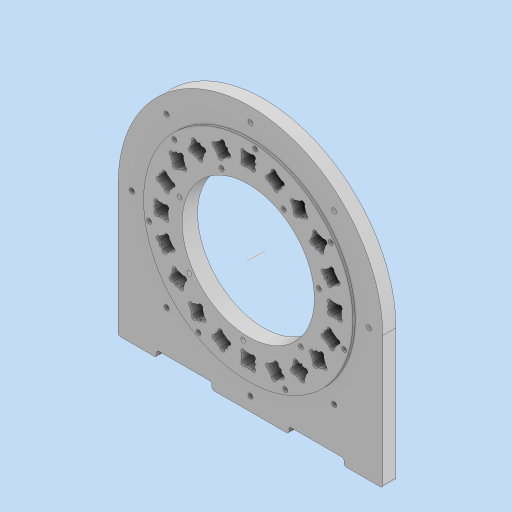
# Autodesk Inventor part: Ring_842
Saved by Autodesk Inventor 2024.2 (Build 282272000, 272)
## iProperties
Created: 2025-04-23
Part Number: Ring_842
Material: Generic
Document SubType Name: Modeling
Designer: 23661194
Density: 1 g/cm^3
Appearance: Default
Author: 23661194
Autodesk Inventor part; units mm, degrees
ref_plane "YZ Plane" through (0, 0, 0) normal (1, 0, 0) x (0, 1, 0)
ref_plane "XZ Plane" through (0, 0, 0) normal (0, 1, 0) x (-1, 0, 0)
ref_plane "XY Plane" through (0, 0, 0) normal (0, 0, 1) x (1, 0, 0)
sketch "Sketch1" plane through (0, 0, 0) normal (0, 0, 1) x (1, 0, 0)
  circle A0 centre (0, 0) radius 60
  circle A1 centre (0, 0) radius 120
  circle A2 centre (0, 0) radius 95
  dimension "d0" = 120
  dimension "d1" = 240
  dimension "d2" = 190
  constraints: 3 centre point, 3 coincident
  measures "d0" diameter of A0
  measures "d1" diameter of A1
  measures "d2" diameter of A2
extrude "Extrusion1" add sketch "Sketch1" along normal blind 12 contours A1 | A2
extrude "Extrusion2" add sketch "Sketch1" along normal blind 14 contours A2
sketch "Sketch3" plane through (0, 0, 14) normal (0, 0, 1) x (1, 0, 0)
  circle A0 centre (0, 0) radius 78.7024
  line L0 (78.7024, 0) -> (0, 0)
  line L1 (74.8504, 24.3204) -> (0, 0)
  line L2 (63.6716, 46.2601) -> (0, 0)
  line L3 (46.2601, 63.6716) -> (0, 0)
  line L4 (24.3204, 74.8504) -> (0, 0)
  line L5 (0, 78.7024) -> (0, 0)
  line L6 (-24.3204, 74.8504) -> (0, 0)
  line L7 (-46.2601, 63.6716) -> (0, 0)
  line L8 (-63.6716, 46.2601) -> (0, 0)
  line L9 (-74.8504, 24.3204) -> (0, 0)
  line L10 (-78.7024, 0) -> (0, 0)
  line L11 (-74.8504, -24.3204) -> (0, 0)
  line L12 (-63.6716, -46.2601) -> (0, 0)
  line L13 (-46.2601, -63.6716) -> (0, 0)
  line L14 (-24.3204, -74.8504) -> (0, 0)
  line L15 (0, -78.7024) -> (0, 0)
  line L16 (24.3204, -74.8504) -> (0, 0)
  line L17 (46.2601, -63.6716) -> (0, 0)
  line L18 (63.6716, -46.2601) -> (0, 0)
  line L19 (74.8504, -24.3204) -> (0, 0)
  line L20 (-168, 0) -> (168, 0) projected
  line L21 (84.6424, 5.94) -> (72.7624, 5.94)
  line L22 (72.7624, 5.94) -> (72.7624, -5.94)
  line L23 (72.7624, -5.94) -> (84.6424, -5.94)
  line L24 (84.6424, -5.94) -> (84.6424, 5.94)
  line L25 (84.6424, 5.94) -> (72.7624, -5.94) construction
  line L26 (72.7624, 5.94) -> (84.6424, -5.94) construction
  circle A1 centre (78.7024, 0) radius 2
  circle A2 centre (74.1754, -4.527) radius 2.1
  circle A3 centre (83.2294, -4.527) radius 2.1
  circle A4 centre (83.2294, 4.527) radius 2.1
  circle A5 centre (74.1754, 4.527) radius 2.1
  circle A6 centre (72.4024, 0) radius 0.75
  line L27 (72.4024, 0) -> (78.7024, 0)
  line L28 (76.1645, 32.6174) -> (66.5534, 25.6345)
  line L29 (66.5534, 25.6345) -> (73.5363, 16.0234)
  line L30 (73.5363, 16.0234) -> (83.1474, 23.0063)
  line L31 (83.1474, 23.0063) -> (76.1645, 32.6174)
  line L32 (76.1645, 32.6174) -> (73.5363, 16.0234) construction
  line L33 (66.5534, 25.6345) -> (83.1474, 23.0063) construction
  circle A7 centre (74.8504, 24.3204) radius 2
  circle A8 centre (73.8489, 17.9971) radius 2.1
  circle A9 centre (81.1737, 23.3189) radius 2.1
  circle A10 centre (75.8519, 30.6437) radius 2.1
  circle A11 centre (68.5271, 25.3219) radius 2.1
  circle A12 centre (69.7536, 20.6173) radius 0.75
  line L34 (69.7536, 20.6173) -> (74.8504, 24.3204)
  line L35 (59.8579, 53.7449) -> (56.1867, 42.4464)
  line L36 (56.1867, 42.4464) -> (67.4853, 38.7753)
  line L37 (67.4853, 38.7753) -> (71.1564, 50.0738)
  line L38 (71.1564, 50.0738) -> (59.8579, 53.7449)
  line L39 (59.8579, 53.7449) -> (67.4853, 38.7753) construction
  line L40 (56.1867, 42.4464) -> (71.1564, 50.0738) construction
  circle A13 centre (63.6716, 46.2601) radius 2
  circle A14 centre (66.5781, 40.5558) radius 2.1
  circle A15 centre (69.3759, 49.1666) radius 2.1
  circle A16 centre (60.7651, 51.9645) radius 2.1
  circle A17 centre (57.9672, 43.3536) radius 2.1
  circle A18 centre (61.7248, 40.2684) radius 0.75
  line L41 (61.7248, 40.2684) -> (63.6716, 46.2601)
  line L42 (38.7753, 67.4853) -> (42.4464, 56.1867)
  line L43 (42.4464, 56.1867) -> (53.7449, 59.8579)
  line L44 (53.7449, 59.8579) -> (50.0738, 71.1564)
  line L45 (50.0738, 71.1564) -> (38.7753, 67.4853)
  line L46 (38.7753, 67.4853) -> (53.7449, 59.8579) construction
  line L47 (42.4464, 56.1867) -> (50.0738, 71.1564) construction
  circle A19 centre (46.2601, 63.6716) radius 2
  circle A20 centre (51.9645, 60.7651) radius 2.1
  circle A21 centre (49.1666, 69.3759) radius 2.1
  circle A22 centre (40.5558, 66.5781) radius 2.1
  circle A23 centre (43.3536, 57.9672) radius 2.1
  circle A24 centre (48.2069, 57.6799) radius 0.75
  line L48 (48.2069, 57.6799) -> (46.2601, 63.6716)
  line L49 (16.0234, 73.5363) -> (25.6345, 66.5534)
  line L50 (25.6345, 66.5534) -> (32.6174, 76.1645)
  line L51 (32.6174, 76.1645) -> (23.0063, 83.1474)
  line L52 (23.0063, 83.1474) -> (16.0234, 73.5363)
  line L53 (16.0234, 73.5363) -> (32.6174, 76.1645) construction
  line L54 (25.6345, 66.5534) -> (23.0063, 83.1474) construction
  circle A25 centre (24.3204, 74.8504) radius 2
  circle A26 centre (30.6437, 75.8519) radius 2.1
  circle A27 centre (23.3189, 81.1737) radius 2.1
  circle A28 centre (17.9971, 73.8489) radius 2.1
  circle A29 centre (25.3219, 68.5271) radius 2.1
  circle A30 centre (29.4172, 71.1474) radius 0.75
  line L55 (29.4172, 71.1474) -> (24.3204, 74.8504)
  line L56 (-5.94, 72.7624) -> (5.94, 72.7624)
  line L57 (5.94, 72.7624) -> (5.94, 84.6424)
  line L58 (5.94, 84.6424) -> (-5.94, 84.6424)
  line L59 (-5.94, 84.6424) -> (-5.94, 72.7624)
  line L60 (-5.94, 72.7624) -> (5.94, 84.6424) construction
  line L61 (5.94, 72.7624) -> (-5.94, 84.6424) construction
  circle A31 centre (0, 78.7024) radius 2
  circle A32 centre (4.527, 83.2294) radius 2.1
  circle A33 centre (-4.527, 83.2294) radius 2.1
  circle A34 centre (-4.527, 74.1754) radius 2.1
  circle A35 centre (4.527, 74.1754) radius 2.1
  circle A36 centre (6.3, 78.7024) radius 0.75
  line L62 (6.3, 78.7024) -> (0, 78.7024)
  line L63 (-25.6345, 66.5534) -> (-16.0234, 73.5363)
  line L64 (-16.0234, 73.5363) -> (-23.0063, 83.1474)
  line L65 (-23.0063, 83.1474) -> (-32.6174, 76.1645)
  line L66 (-32.6174, 76.1645) -> (-25.6345, 66.5534)
  line L67 (-25.6345, 66.5534) -> (-23.0063, 83.1474) construction
  line L68 (-16.0234, 73.5363) -> (-32.6174, 76.1645) construction
  circle A37 centre (-24.3204, 74.8504) radius 2
  circle A38 centre (-23.3189, 81.1737) radius 2.1
  circle A39 centre (-30.6437, 75.8519) radius 2.1
  circle A40 centre (-25.3219, 68.5271) radius 2.1
  circle A41 centre (-17.9971, 73.8489) radius 2.1
  circle A42 centre (-19.2236, 78.5535) radius 0.75
  line L69 (-19.2236, 78.5535) -> (-24.3204, 74.8504)
  line L70 (-42.4464, 56.1867) -> (-38.7753, 67.4853)
  line L71 (-38.7753, 67.4853) -> (-50.0738, 71.1564)
  line L72 (-50.0738, 71.1564) -> (-53.7449, 59.8579)
  line L73 (-53.7449, 59.8579) -> (-42.4464, 56.1867)
  line L74 (-42.4464, 56.1867) -> (-50.0738, 71.1564) construction
  line L75 (-38.7753, 67.4853) -> (-53.7449, 59.8579) construction
  circle A43 centre (-46.2601, 63.6716) radius 2
  circle A44 centre (-49.1666, 69.3759) radius 2.1
  circle A45 centre (-51.9645, 60.7651) radius 2.1
  circle A46 centre (-43.3536, 57.9672) radius 2.1
  circle A47 centre (-40.5558, 66.5781) radius 2.1
  circle A48 centre (-44.3133, 69.6632) radius 0.75
  line L76 (-44.3133, 69.6632) -> (-46.2601, 63.6716)
  line L77 (-56.1867, 42.4464) -> (-59.8579, 53.7449)
  line L78 (-59.8579, 53.7449) -> (-71.1564, 50.0738)
  line L79 (-71.1564, 50.0738) -> (-67.4853, 38.7753)
  line L80 (-67.4853, 38.7753) -> (-56.1867, 42.4464)
  line L81 (-56.1867, 42.4464) -> (-71.1564, 50.0738) construction
  line L82 (-59.8579, 53.7449) -> (-67.4853, 38.7753) construction
  circle A49 centre (-63.6716, 46.2601) radius 2
  circle A50 centre (-69.3759, 49.1666) radius 2.1
  circle A51 centre (-66.5781, 40.5558) radius 2.1
  circle A52 centre (-57.9672, 43.3536) radius 2.1
  circle A53 centre (-60.7651, 51.9645) radius 2.1
  circle A54 centre (-65.6184, 52.2518) radius 0.75
  line L83 (-65.6184, 52.2518) -> (-63.6716, 46.2601)
  line L84 (-66.5534, 25.6345) -> (-76.1645, 32.6174)
  line L85 (-76.1645, 32.6174) -> (-83.1474, 23.0063)
  line L86 (-83.1474, 23.0063) -> (-73.5363, 16.0234)
  line L87 (-73.5363, 16.0234) -> (-66.5534, 25.6345)
  line L88 (-66.5534, 25.6345) -> (-83.1474, 23.0063) construction
  line L89 (-76.1645, 32.6174) -> (-73.5363, 16.0234) construction
  circle A55 centre (-74.8504, 24.3204) radius 2
  circle A56 centre (-81.1737, 23.3189) radius 2.1
  circle A57 centre (-73.8489, 17.9971) radius 2.1
  circle A58 centre (-68.5271, 25.3219) radius 2.1
  circle A59 centre (-75.8519, 30.6437) radius 2.1
  circle A60 centre (-79.9472, 28.0234) radius 0.75
  line L90 (-79.9472, 28.0234) -> (-74.8504, 24.3204)
  line L91 (-72.7624, 5.94) -> (-84.6424, 5.94)
  line L92 (-84.6424, 5.94) -> (-84.6424, -5.94)
  line L93 (-84.6424, -5.94) -> (-72.7624, -5.94)
  line L94 (-72.7624, -5.94) -> (-72.7624, 5.94)
  line L95 (-72.7624, 5.94) -> (-84.6424, -5.94) construction
  line L96 (-84.6424, 5.94) -> (-72.7624, -5.94) construction
  circle A61 centre (-78.7024, 0) radius 2
  circle A62 centre (-83.2294, -4.527) radius 2.1
  circle A63 centre (-74.1754, -4.527) radius 2.1
  circle A64 centre (-74.1754, 4.527) radius 2.1
  circle A65 centre (-83.2294, 4.527) radius 2.1
  circle A66 centre (-85.0024, 0) radius 0.75
  line L97 (-85.0024, 0) -> (-78.7024, 0)
  line L98 (-73.5363, -16.0234) -> (-83.1474, -23.0063)
  line L99 (-83.1474, -23.0063) -> (-76.1645, -32.6174)
  line L100 (-76.1645, -32.6174) -> (-66.5534, -25.6345)
  line L101 (-66.5534, -25.6345) -> (-73.5363, -16.0234)
  line L102 (-73.5363, -16.0234) -> (-76.1645, -32.6174) construction
  line L103 (-83.1474, -23.0063) -> (-66.5534, -25.6345) construction
  circle A67 centre (-74.8504, -24.3204) radius 2
  circle A68 centre (-75.8519, -30.6437) radius 2.1
  circle A69 centre (-68.5271, -25.3219) radius 2.1
  circle A70 centre (-73.8489, -17.9971) radius 2.1
  circle A71 centre (-81.1737, -23.3189) radius 2.1
  circle A72 centre (-79.9472, -28.0234) radius 0.75
  line L104 (-79.9472, -28.0234) -> (-74.8504, -24.3204)
  line L105 (-67.4853, -38.7753) -> (-71.1564, -50.0738)
  line L106 (-71.1564, -50.0738) -> (-59.8579, -53.7449)
  line L107 (-59.8579, -53.7449) -> (-56.1867, -42.4464)
  line L108 (-56.1867, -42.4464) -> (-67.4853, -38.7753)
  line L109 (-67.4853, -38.7753) -> (-59.8579, -53.7449) construction
  line L110 (-71.1564, -50.0738) -> (-56.1867, -42.4464) construction
  circle A73 centre (-63.6716, -46.2601) radius 2
  circle A74 centre (-60.7651, -51.9645) radius 2.1
  circle A75 centre (-57.9672, -43.3536) radius 2.1
  circle A76 centre (-66.5781, -40.5558) radius 2.1
  circle A77 centre (-69.3759, -49.1666) radius 2.1
  circle A78 centre (-65.6184, -52.2518) radius 0.75
  line L111 (-65.6184, -52.2518) -> (-63.6716, -46.2601)
  line L112 (-53.7449, -59.8579) -> (-50.0738, -71.1564)
  line L113 (-50.0738, -71.1564) -> (-38.7753, -67.4853)
  line L114 (-38.7753, -67.4853) -> (-42.4464, -56.1867)
  line L115 (-42.4464, -56.1867) -> (-53.7449, -59.8579)
  line L116 (-53.7449, -59.8579) -> (-38.7753, -67.4853) construction
  line L117 (-50.0738, -71.1564) -> (-42.4464, -56.1867) construction
  circle A79 centre (-46.2601, -63.6716) radius 2
  circle A80 centre (-40.5558, -66.5781) radius 2.1
  circle A81 centre (-43.3536, -57.9672) radius 2.1
  circle A82 centre (-51.9645, -60.7651) radius 2.1
  circle A83 centre (-49.1666, -69.3759) radius 2.1
  circle A84 centre (-44.3133, -69.6632) radius 0.75
  line L118 (-44.3133, -69.6632) -> (-46.2601, -63.6716)
  line L119 (-32.6174, -76.1645) -> (-23.0063, -83.1474)
  line L120 (-23.0063, -83.1474) -> (-16.0234, -73.5363)
  line L121 (-16.0234, -73.5363) -> (-25.6345, -66.5534)
  line L122 (-25.6345, -66.5534) -> (-32.6174, -76.1645)
  line L123 (-32.6174, -76.1645) -> (-16.0234, -73.5363) construction
  line L124 (-23.0063, -83.1474) -> (-25.6345, -66.5534) construction
  circle A85 centre (-24.3204, -74.8504) radius 2
  circle A86 centre (-17.9971, -73.8489) radius 2.1
  circle A87 centre (-25.3219, -68.5271) radius 2.1
  circle A88 centre (-30.6437, -75.8519) radius 2.1
  circle A89 centre (-23.3189, -81.1737) radius 2.1
  circle A90 centre (-19.2236, -78.5535) radius 0.75
  line L125 (-19.2236, -78.5535) -> (-24.3204, -74.8504)
  line L126 (-5.94, -84.6424) -> (5.94, -84.6424)
  line L127 (5.94, -84.6424) -> (5.94, -72.7624)
  line L128 (5.94, -72.7624) -> (-5.94, -72.7624)
  line L129 (-5.94, -72.7624) -> (-5.94, -84.6424)
  line L130 (-5.94, -84.6424) -> (5.94, -72.7624) construction
  line L131 (5.94, -84.6424) -> (-5.94, -72.7624) construction
  circle A91 centre (0, -78.7024) radius 2
  circle A92 centre (4.527, -74.1754) radius 2.1
  circle A93 centre (-4.527, -74.1754) radius 2.1
  circle A94 centre (-4.527, -83.2294) radius 2.1
  circle A95 centre (4.527, -83.2294) radius 2.1
  circle A96 centre (6.3, -78.7024) radius 0.75
  line L132 (6.3, -78.7024) -> (0, -78.7024)
  line L133 (23.0063, -83.1474) -> (32.6174, -76.1645)
  line L134 (32.6174, -76.1645) -> (25.6345, -66.5534)
  line L135 (25.6345, -66.5534) -> (16.0234, -73.5363)
  line L136 (16.0234, -73.5363) -> (23.0063, -83.1474)
  line L137 (23.0063, -83.1474) -> (25.6345, -66.5534) construction
  line L138 (32.6174, -76.1645) -> (16.0234, -73.5363) construction
  circle A97 centre (24.3204, -74.8504) radius 2
  circle A98 centre (25.3219, -68.5271) radius 2.1
  circle A99 centre (17.9971, -73.8489) radius 2.1
  circle A100 centre (23.3189, -81.1737) radius 2.1
  circle A101 centre (30.6437, -75.8519) radius 2.1
  circle A102 centre (29.4172, -71.1474) radius 0.75
  line L139 (29.4172, -71.1474) -> (24.3204, -74.8504)
  line L140 (83.1474, -23.0063) -> (73.5363, -16.0234)
  line L141 (73.5363, -16.0234) -> (66.5534, -25.6345)
  line L142 (66.5534, -25.6345) -> (76.1645, -32.6174)
  line L143 (76.1645, -32.6174) -> (83.1474, -23.0063)
  line L144 (83.1474, -23.0063) -> (66.5534, -25.6345) construction
  line L145 (73.5363, -16.0234) -> (76.1645, -32.6174) construction
  circle A103 centre (74.8504, -24.3204) radius 2
  circle A104 centre (68.5271, -25.3219) radius 2.1
  circle A105 centre (75.8519, -30.6437) radius 2.1
  circle A106 centre (81.1737, -23.3189) radius 2.1
  circle A107 centre (73.8489, -17.9971) radius 2.1
  circle A108 centre (69.7536, -20.6173) radius 0.75
  line L146 (69.7536, -20.6173) -> (74.8504, -24.3204)
  line L147 (50.0738, -71.1564) -> (53.7449, -59.8579)
  line L148 (53.7449, -59.8579) -> (42.4464, -56.1867)
  line L149 (42.4464, -56.1867) -> (38.7753, -67.4853)
  line L150 (38.7753, -67.4853) -> (50.0738, -71.1564)
  line L151 (50.0738, -71.1564) -> (42.4464, -56.1867) construction
  line L152 (53.7449, -59.8579) -> (38.7753, -67.4853) construction
  circle A109 centre (46.2601, -63.6716) radius 2
  circle A110 centre (43.3536, -57.9672) radius 2.1
  circle A111 centre (40.5558, -66.5781) radius 2.1
  circle A112 centre (49.1666, -69.3759) radius 2.1
  circle A113 centre (51.9645, -60.7651) radius 2.1
  circle A114 centre (48.2069, -57.6799) radius 0.75
  line L153 (48.2069, -57.6799) -> (46.2601, -63.6716)
  line L154 (71.1564, -50.0738) -> (67.4853, -38.7753)
  line L155 (67.4853, -38.7753) -> (56.1867, -42.4464)
  line L156 (56.1867, -42.4464) -> (59.8579, -53.7449)
  line L157 (59.8579, -53.7449) -> (71.1564, -50.0738)
  line L158 (71.1564, -50.0738) -> (56.1867, -42.4464) construction
  line L159 (67.4853, -38.7753) -> (59.8579, -53.7449) construction
  circle A115 centre (63.6716, -46.2601) radius 2
  circle A116 centre (57.9672, -43.3536) radius 2.1
  circle A117 centre (60.7651, -51.9645) radius 2.1
  circle A118 centre (69.3759, -49.1666) radius 2.1
  circle A119 centre (66.5781, -40.5558) radius 2.1
  circle A120 centre (61.7248, -40.2684) radius 0.75
  line L160 (61.7248, -40.2684) -> (63.6716, -46.2601)
  point P0 (73.7646, -30.8737)
  point P1 (77.9082, -30.2174)
  point P2 (81.4037, -25.4062)
  point P3 (80.7475, -21.2626)
  point P4 (75.9363, -17.767)
  point P5 (71.7926, -18.4233)
  point P6 (68.2971, -23.2345)
  point P7 (68.9534, -27.3782)
  point P8 (57.1034, -45.2677)
  point P9 (58.9412, -50.9236)
  point P10 (62.6792, -52.8282)
  point P11 (68.3351, -50.9905)
  point P12 (70.2397, -47.2525)
  point P13 (68.402, -41.5966)
  point P14 (64.664, -39.692)
  point P15 (59.0081, -41.5297)
  point P16 (39.692, -64.664)
  point P17 (41.5966, -68.402)
  point P18 (47.2525, -70.2397)
  point P19 (50.9905, -68.3351)
  point P20 (52.8282, -62.6792)
  point P21 (50.9236, -58.9412)
  point P22 (45.2677, -57.1034)
  point P23 (41.5297, -59.0081)
  point P24 (17.767, -75.9363)
  point P25 (21.2626, -80.7475)
  point P26 (25.4062, -81.4037)
  point P27 (30.2174, -77.9082)
  point P28 (30.8737, -73.7646)
  point P29 (27.3782, -68.9534)
  point P30 (23.2345, -68.2971)
  point P31 (18.4233, -71.7926)
  point P32 (5.94, -75.7289)
  point P33 (2.9735, -72.7624)
  point P34 (-2.9735, -72.7624)
  point P35 (-5.94, -75.7289)
  point P36 (-5.94, -81.6759)
  point P37 (-2.9735, -84.6424)
  point P38 (2.9735, -84.6424)
  point P39 (5.94, -81.6759)
  point P40 (-23.2345, -68.2971)
  point P41 (-27.3782, -68.9534)
  point P42 (-30.8737, -73.7646)
  point P43 (-30.2174, -77.9082)
  point P44 (-25.4062, -81.4037)
  point P45 (-21.2626, -80.7475)
  point P46 (-17.767, -75.9363)
  point P47 (-18.4233, -71.7926)
  point P48 (-52.8282, -62.6792)
  point P49 (-50.9905, -68.3351)
  point P50 (-47.2525, -70.2397)
  point P51 (-41.5966, -68.402)
  point P52 (-39.692, -64.664)
  point P53 (-41.5297, -59.0081)
  point P54 (-45.2677, -57.1034)
  point P55 (-50.9236, -58.9412)
  point P56 (-58.9412, -50.9236)
  point P57 (-57.1034, -45.2677)
  point P58 (-59.0081, -41.5297)
  point P59 (-64.664, -39.692)
  point P60 (-68.402, -41.5966)
  point P61 (-70.2397, -47.2525)
  point P62 (-68.3351, -50.9905)
  point P63 (-62.6792, -52.8282)
  point P64 (-71.7926, -18.4233)
  point P65 (-75.9363, -17.767)
  point P66 (-80.7475, -21.2626)
  point P67 (-81.4037, -25.4062)
  point P68 (-77.9082, -30.2174)
  point P69 (-73.7646, -30.8737)
  point P70 (-68.9534, -27.3782)
  point P71 (-68.2971, -23.2345)
  point P72 (-72.7624, 2.9735)
  point P73 (-75.7289, 5.94)
  point P74 (-81.6759, 5.94)
  point P75 (-84.6424, 2.9735)
  point P76 (-84.6424, -2.9735)
  point P77 (-81.6759, -5.94)
  point P78 (-75.7289, -5.94)
  point P79 (-72.7624, -2.9735)
  point P80 (-68.2971, 23.2345)
  point P81 (-68.9534, 27.3782)
  point P82 (-73.7646, 30.8737)
  point P83 (-77.9082, 30.2174)
  point P84 (-81.4037, 25.4062)
  point P85 (-80.7475, 21.2626)
  point P86 (-75.9363, 17.767)
  point P87 (-71.7926, 18.4233)
  point P88 (-59.0081, 41.5297)
  point P89 (-57.1034, 45.2677)
  point P90 (-58.9412, 50.9236)
  point P91 (-62.6792, 52.8282)
  point P92 (-68.3351, 50.9905)
  point P93 (-70.2397, 47.2525)
  point P94 (-68.402, 41.5966)
  point P95 (-64.664, 39.692)
  point P96 (-45.2677, 57.1034)
  point P97 (-41.5297, 59.0081)
  point P98 (-39.692, 64.664)
  point P99 (-41.5966, 68.402)
  point P100 (-47.2525, 70.2397)
  point P101 (-50.9905, 68.3351)
  point P102 (-52.8282, 62.6792)
  point P103 (-50.9236, 58.9412)
  point P104 (-18.4233, 71.7926)
  point P105 (-17.767, 75.9363)
  point P106 (-21.2626, 80.7475)
  point P107 (-25.4062, 81.4037)
  point P108 (-30.2174, 77.9082)
  point P109 (-30.8737, 73.7646)
  point P110 (-27.3782, 68.9534)
  point P111 (-23.2345, 68.2971)
  point P112 (-5.94, 75.7289)
  point P113 (-2.9735, 72.7624)
  point P114 (2.9735, 72.7624)
  point P115 (5.94, 75.7289)
  point P116 (5.94, 81.6759)
  point P117 (2.9735, 84.6424)
  point P118 (-2.9735, 84.6424)
  point P119 (-5.94, 81.6759)
  point P120 (17.767, 75.9363)
  point P121 (18.4233, 71.7926)
  point P122 (23.2345, 68.2971)
  point P123 (27.3782, 68.9534)
  point P124 (30.8737, 73.7646)
  point P125 (30.2174, 77.9082)
  point P126 (25.4062, 81.4037)
  point P127 (21.2626, 80.7475)
  point P128 (39.692, 64.664)
  point P129 (41.5297, 59.0081)
  point P130 (45.2677, 57.1034)
  point P131 (50.9236, 58.9412)
  point P132 (52.8282, 62.6792)
  point P133 (50.9905, 68.3351)
  point P134 (47.2525, 70.2397)
  point P135 (41.5966, 68.402)
  point P136 (68.402, 41.5966)
  point P137 (70.2397, 47.2525)
  point P138 (68.3351, 50.9905)
  point P139 (62.6792, 52.8282)
  point P140 (58.9412, 50.9236)
  point P141 (57.1034, 45.2677)
  point P142 (59.0081, 41.5297)
  point P143 (64.664, 39.692)
  point P144 (68.9534, 27.3782)
  point P145 (68.2971, 23.2345)
  point P146 (71.7926, 18.4233)
  point P147 (75.9363, 17.767)
  point P148 (80.7475, 21.2626)
  point P149 (81.4037, 25.4062)
  point P150 (77.9082, 30.2174)
  point P151 (73.7646, 30.8737)
  point P152 (75.7289, 5.94)
  point P153 (72.7624, 2.9735)
  point P154 (72.7624, -2.9735)
  point P155 (75.7289, -5.94)
  point P156 (81.6759, -5.94)
  point P157 (84.6424, -2.9735)
  point P158 (84.6424, 2.9735)
  point P159 (81.6759, 5.94)
  dimension "d61" = 157.4048
  dimension "d67" = -36
  dimension "d68" = -72
  dimension "d69" = -108
  dimension "d70" = -144
  dimension "d71" = -180
  dimension "d72" = -216
  dimension "d73" = -252
  dimension "d74" = -288
  dimension "d75" = -324
  dimension "d76" = 0
  dimension "d77" = -36
  dimension "d78" = -72
  dimension "d79" = -108
  dimension "d80" = -144
  dimension "d81" = -180
  dimension "d82" = -216
  dimension "d83" = -252
  dimension "d84" = -288
  dimension "d85" = -324
  dimension "d64" = 360
  dimension "d66" = 0
  constraints: 40 end point, 1 coincident, 1 horizontal, 1 horizontal alignment, 84 other
  measures "d66" vertical extent of L0
extrude "Extrusion3" cut sketch "Sketch3" against normal blind 12 contours L0 A1 A0 | L20 A1 A0 | A0 A1 L0 | A0 A1 L20 | A1 L0 A6 L22 A5 L21 A0 | A0 L21 A4 L24 L20 A1 | A1 L20 L24 A3 L23 A0 | A0 L23 A2 L22 A6 L0 A1 | A6 L22 L0 | L0 L22 A6 | L30 A8 L29 A12 L34 A7 A0 | A0 A7 L28 A10 L31 A9 L30 | A4 L24 L21 | L21 L24 A4 | A5 L22 L21 | L21 L22 A5 | L140 A106 L143 A105 L142 A0 A103 | A0 A103 L146 A108 L141 A107 L140 | A2 L22 L23 | L23 L22 A2 | A3 L24 L23 | L23 L24 A3 | A7 L34 A0 | A0 A7 | A8 L29 L30 | L30 L29 A8 | A9 L31 L30 | L30 L31 A9 | A103 A0 | A0 L146 A103 | A106 L143 L140 | L140 L143 A106 | A107 L141 L140 | L140 L141 A107 | L1 A7 A0 | L34 A7 L1 | L34 A12 L29 L1 A7 | A0 A103 L19 | L19 A103 L146 | A103 L19 L141 A108 L146 | A7 L1 L29 A11 L28 A0 | L34 L29 A12 | A12 L29 L34 | A10 L28 L31 | L31 L28 A10 | A0 L142 A104 L141 L19 A103 | L146 L141 A108 | A108 L141 L146 | A105 L142 L143 | L143 L142 A105 | A17 L35 L36 L2 | L2 L36 A17 | A23 L42 L3 | L3 L42 L43 A23 | L49 A28 L52 A0 A25 L4 | L4 A25 L55 A30 L50 A29 L49 | L56 A34 L59 A0 A31 L5 | L5 A31 A0 A36 L57 A35 L56 | L63 A40 L66 A0 A37 L6 | L6 A37 A0 L64 A41 L63 | A46 L73 L70 L7 | L7 L70 A46 | A52 L80 L8 | L8 L80 L77 A52 | L87 A57 L86 A0 A55 L9 | L9 A55 A0 L84 A58 L87 | L94 A63 L93 A0 A61 L10 | L10 A61 A0 L91 A64 L94 | L101 A69 L100 A0 A67 L11 | L11 A67 A0 L98 A70 L101 | A75 L107 L108 L12 | L12 L108 A75 | A81 L114 L13 | L13 L114 L115 A81 | L121 A86 L120 A0 A85 L14 | L14 A85 A0 L122 A87 L121 | L128 A92 L127 A96 A0 A91 L15 | L15 A91 A0 L129 A93 L128 | L135 A98 L134 A102 L139 A97 L16 | L16 A97 A0 L136 A99 L135 | A110 L148 L149 L17 | L17 L149 A110 | A116 L155 L18 | L18 L155 L156 A116 | A11 L28 L29 | L29 L28 A11 | L36 L35 A17 L2 | L2 A17 L36 | L35 A16 A0 A13 L2 A17 | A17 L2 A13 L41 A18 L36 | L42 A23 L3 | L3 A23 L43 L42 | L42 A22 A0 A19 L3 A23 | A23 L3 A19 L48 A24 L43 | A25 A0 L4 | L4 L55 A25 | A28 L52 L49 | L49 L52 A28 | A29 L50 L49 | L49 L50 A29 | A31 A0 L5 | L5 A0 A31 | A34 L59 L56 | L56 L59 A34 | A35 L57 L56 | L56 L57 A35 | A37 A0 L6 | L6 A0 A37 | A40 L66 L63 | L63 L66 A40 | A41 L64 L63 | L63 L64 A41 | L70 L73 A46 L7 | L7 A46 L70 | L73 A45 A0 A43 L7 A46 | L80 A52 L8 | L8 A52 L77 L80 | L80 A51 A0 A49 L8 A52 | A55 A0 L9 | L9 A0 A55 | A57 L86 L87 | L87 L86 A57 | A58 L84 L87 | L87 L84 A58 | A61 A0 L10 | L10 A0 A61 | A63 L93 L94 | L94 L93 A63 | A64 L91 L94 | L94 L91 A64 | A67 A0 L11 | L11 A0 A67 | A69 L100 L101 | L101 L100 A69 | A70 L98 L101 | L101 L98 A70 | L108 L107 A75 L12 | L12 A75 L108 | A75 L12 A73 A0 A76 L108 | L114 A81 L13 | L13 A81 L115 L114 | A81 L13 A79 A0 A82 L115 | A85 A0 L14 | L14 A0 A85 | A86 L120 L121 | L121 L120 A86 | A87 L122 L121 | L121 L122 A87 | A91 A0 L15 | L15 A0 A91 | A92 L127 L128 | L128 L127 A92 | A93 L129 L128 | L128 L129 A93 | A97 L139 L16 | L16 A0 A97 | A98 L134 L135 | L135 L134 A98 | A99 L136 L135 | L135 L136 A99 | L149 L148 A110 L17 | L17 A110 L149 | L148 A114 L153 A109 L17 A110 | A110 L17 A109 A0 A111 L149 | L155 A116 L18 | L18 A116 L156 L155 | L155 A120 L160 A115 L18 A116 | A116 L18 A115 A0 A117 L156 | A104 L142 L141 | L141 L142 A104 | A14 L36 L37 A0 | A0 L37 A14 | A119 L154 A0 | A0 L154 L155 A119 | A16 A0 L35 | L35 A0 A16 | A18 L41 L36 | A22 A0 L45 L42 | L42 L45 A0 A22 | A24 L48 L43 | A0 A25 | A0 A25 L55 | A0 L52 A27 L51 A26 L50 A25 | A25 A0 L50 A30 L55 | L62 A31 A0 | A0 A31 L62 | A0 L59 A33 L58 A32 L57 A36 L62 A31 | A31 L62 A36 A0 | L69 A37 A0 | A0 A37 L69 | A0 L66 A39 L65 A38 L64 A42 L69 A37 | L7 A43 A0 A47 L70 A46 | A45 A0 L73 | L73 A0 A45 | L8 A49 A0 A53 L77 A52 | A51 A0 L79 L80 | L80 L79 A0 A51 | L90 A55 A0 | A0 A55 L90 | A0 L86 A56 L85 A60 L90 A55 | L20 A61 A0 | A0 A61 L20 | A61 L20 A66 L92 A65 L91 A0 | A0 L93 A62 L92 A66 L20 A61 | L104 A67 A0 | A0 A67 L104 | A67 L104 A72 L99 A71 L98 A0 | A75 L107 A74 A0 A73 L12 | A76 A0 L105 L108 | L108 L105 A0 A76 | A81 L114 A80 A0 A79 L13 | A82 A0 L115 | L115 A0 A82 | L125 A85 A0 | A0 A85 L125 | A85 L125 A90 L120 A89 L119 A88 L122 A0 | L132 A91 A0 | A0 A91 L132 | A0 A96 L132 A91 | A91 L132 A96 L127 A95 L126 A94 L129 A0 | A0 A97 | L139 A97 A0 | L139 A102 L134 A0 A97 | A97 A0 L134 A101 L133 A100 L136 | L148 L153 A114 | A111 A0 L150 L149 | L149 L150 A0 A111 | L155 L160 A120 | A117 A0 L156 | L156 A0 A117 | L37 L36 A14 A0 | A0 A14 L37 | L36 A18 L41 A13 A0 A14 | L154 A119 A0 | A0 A119 L155 L154 | A119 A0 A115 L160 A120 L155 | A13 A0 L2 | L2 L41 A13 | L35 L38 A16 A0 | A0 A16 L38 L35 | A16 L38 A15 L37 A14 A0 A13 | L41 A18 L36 | A19 A0 L3 | L3 L48 A19 | A22 L45 A0 | A22 L45 A21 L44 A20 A0 A19 | A0 L45 A22 | L48 A24 L43 | L48 A19 A0 A20 L43 A24 | L55 L50 A30 | A30 L50 L55 | A36 L62 L57 A0 | A0 L57 A36 | A37 L69 A42 L64 A0 | A43 A0 L7 | L7 A0 A43 | A47 A0 L71 L70 | L70 L71 A0 A47 | L73 L72 A45 A0 | A0 A45 L72 L73 | A49 A0 L8 | L8 A0 A49 | A51 L79 A0 | A53 A0 L77 | L77 A0 A53 | A55 L90 A60 L85 A59 L84 A0 | A0 L100 A68 L99 A72 L104 A67 | A73 A0 L12 | L12 A0 A73 | A74 A0 L107 | L107 A0 A74 | A0 L105 A76 | A79 A0 L13 | L13 A0 A79 | A80 A0 L113 L114 | L114 L113 A0 A80 | L115 L112 A82 A0 | A0 A82 L112 L115 | A0 L120 A90 L125 A85 | A96 L127 A0 | A0 L127 L132 A96 | L139 L134 A102 | A102 L134 L139 | A109 L153 L17 | L17 A0 A109 | L148 A114 L153 | A114 L148 A113 A0 A109 L153 | A111 L150 A0 | A0 A109 A113 L147 A112 L150 A111 | A0 L150 A111 | A115 L160 L18 | L18 A0 A115 | L155 A120 L160 | L156 L157 A117 A0 | A0 A117 L157 L156 | A0 A115 A119 L154 A118 L157 A117 | A0 A13 | A0 A13 L41 | A20 L43 A0 | A0 L43 L44 A20 | A0 A19 | A0 A19 L48 | A27 L51 L52 | L52 L51 A27 | A36 L57 L62 | A33 L58 L59 | L59 L58 A33 | L69 L64 A42 | A42 L64 L69 | A0 L71 A47 | A39 L65 L66 | L66 L65 A39 | L76 A43 A0 | A0 A43 L76 | A0 A45 L72 A44 L71 A48 L76 A43 | A47 L71 A0 | A0 A43 L76 A48 L71 A47 | A0 L77 L78 A53 | L83 A49 A0 | A0 A49 L83 | A0 A51 L79 A50 L78 A54 L83 A49 | L79 A51 A0 | A0 A53 L78 L77 | A0 A49 L83 A54 L78 A53 | L90 L85 A60 | A60 L85 L90 | A56 L85 L86 | L86 L85 A56 | A59 L85 L84 | L84 L85 A59 | A66 L92 L20 | L20 L92 A66 | A65 L92 L91 | L91 L92 A65 | A62 L92 L93 | L93 L92 A62 | L104 L99 A72 | A72 L99 L104 | A71 L99 L98 | L98 L99 A71 | A68 L99 L100 | L100 L99 A68 | L111 A73 A0 | A0 A73 L111 | A73 L111 A78 L106 A77 L105 A76 A0 | L107 L106 A74 A0 | A0 A74 L106 L107 | A74 L106 A78 L111 A73 A0 | A0 A76 L105 | L118 A79 A0 | A0 A79 L118 | A79 L118 A84 L113 A83 L112 A82 A0 | A80 L113 A84 L118 A79 A0 | A0 L113 A80 | L125 L120 A90 | A90 L120 L125 | A80 L113 A0 | A88 L119 L122 | L122 L119 A88 | L132 L127 A96 | A94 L126 L129 | L129 L126 A94 | A100 L133 L136 | L136 L133 A100 | A0 A109 | L153 A109 A0 | A0 A115 | L160 A115 A0 | A113 L147 L148 A0 | A0 L148 A113 | A15 L38 L37 | L37 L38 A15 | A118 L157 L154 | L154 L157 A118 | L43 A20 A0 | A0 A20 L44 L43 | A26 L51 L50 | L50 L51 A26 | A21 L44 L45 | L45 L44 A21 | A44 L71 L72 | L72 L71 A44 | A50 L78 L79 | L79 L78 A50 | A77 L106 L105 | L105 L106 A77 | A83 L113 L112 | L112 L113 A83 | A101 L133 L134 | L134 L133 A101 | L148 A0 A113 | A112 L147 L150 | L150 L147 A112 | L148 L147 A113 A0 | A32 L58 L57 | L57 L58 A32 | A38 L65 L64 | L64 L65 A38 | A48 L76 L71 | A48 L71 L76 | A54 L83 L78 | A54 L78 L83 | L111 L106 A78 | A78 L106 L111 | L118 L113 A84 | A84 L113 L118 | A89 L119 L120 | L120 L119 A89 | A95 L126 L127 | L127 L126 A95 picked at (72.8062, -0.4081) picked at (72.8062, 0.4081) picked at (5.8987, 78.2173) picked at (5.8987, -78.2173) picked at (-84.5986, -0.4081) picked at (-84.5986, 0.4081)
extrude "Extrusion4" cut sketch "Sketch3" against normal blind 2 contours A6 L22 L0 | L0 L22 A6 | L22 A6 L0 | L0 A6 L22 | L34 L29 A12 | A12 L29 L34 | A12 L29 | L146 L141 A108 | A108 L141 L146 | L141 A108 | A18 L41 L36 | L36 A18 | A24 L48 L43 | L43 A24 | A114 L148 | L148 L153 A114 | A120 L155 | L155 L160 A120 | L41 A18 L36 | L48 A24 L43 | L55 L50 A30 | A30 L50 L55 | L50 A30 | A36 L62 L57 A0 | A0 L57 A36 | L57 A0 A36 | A96 L127 A0 | A0 L127 L132 A96 | A96 A0 L127 | L139 L134 A102 | A102 L134 L139 | A102 L134 | L148 A114 L153 | L155 A120 L160 | A0 L57 A36 | A36 L57 L62 | L69 L64 A42 | A42 L64 L69 | L64 A42 | L90 L85 A60 | A60 L85 L90 | A66 L92 L20 | L20 L92 A66 | L104 L99 A72 | A72 L99 L104 | L125 L120 A90 | A90 L120 L125 | A90 L120 | L132 L127 A96 | A0 A96 L127 | A60 L85 | L92 A66 L20 | L20 A66 L92 | L99 A72 | A48 L76 L71 | L71 A48 | A48 L71 L76 | A54 L83 L78 | L78 A54 | A54 L78 L83 | L111 L106 A78 | A78 L106 L111 | A78 L106 | L118 L113 A84 | A84 L113 L118 | A84 L113
extrude "Extrusion5" cut sketch "Sketch3" against normal through all contours L0 A1 A0 | L20 A1 A0 | A0 A1 L0 | A0 A1 L20 | A7 L34 A0 | A0 A7 | A103 A0 | A0 L146 A103 | L1 A7 A0 | L34 A7 L1 | A0 A103 L19 | L19 A103 L146 | A25 A0 L4 | L4 L55 A25 | A31 A0 L5 | L5 A0 A31 | A37 A0 L6 | L6 A0 A37 | A55 A0 L9 | L9 A0 A55 | A61 A0 L10 | L10 A0 A61 | A67 A0 L11 | L11 A0 A67 | A85 A0 L14 | L14 A0 A85 | A91 A0 L15 | L15 A0 A91 | A97 L139 L16 | L16 A0 A97 | A0 A25 | A0 A25 L55 | L62 A31 A0 | A0 A31 L62 | L69 A37 A0 | A0 A37 L69 | L90 A55 A0 | A0 A55 L90 | L20 A61 A0 | A0 A61 L20 | L104 A67 A0 | A0 A67 L104 | L125 A85 A0 | A0 A85 L125 | L132 A91 A0 | A0 A91 L132 | A0 A97 | L139 A97 A0 | A13 A0 L2 | L2 L41 A13 | A19 A0 L3 | L3 L48 A19 | A43 A0 L7 | L7 A0 A43 | A49 A0 L8 | L8 A0 A49 | A73 A0 L12 | L12 A0 A73 | A79 A0 L13 | L13 A0 A79 | A109 L153 L17 | L17 A0 A109 | A115 L160 L18 | L18 A0 A115 | A0 A13 | A0 A13 L41 | A0 A19 | A0 A19 L48 | L76 A43 A0 | A0 A43 L76 | L83 A49 A0 | A0 A49 L83 | L111 A73 A0 | A0 A73 L111 | L118 A79 A0 | A0 A79 L118 | A0 A109 | L153 A109 A0 | A0 A115 | L160 A115 A0
sketch "Sketch4" plane through (0, 0, 12) normal (0, 0, 1) x (1, 0, 0)
  circle A0 centre (0, 0) radius 107.5
  circle A1 centre (0, 107.5) radius 2.15
  circle A2 centre (-76.014, 76.014) radius 2.15
  circle A3 centre (-107.5, 0) radius 2.15
  circle A4 centre (-76.014, -76.014) radius 2.15
  circle A5 centre (0, -107.5) radius 2.15
  circle A6 centre (76.014, -76.014) radius 2.15
  circle A7 centre (107.5, 0) radius 2.15
  circle A8 centre (76.014, 76.014) radius 2.15
  circle A9 centre (0, 0) radius 100
  circle A10 centre (0, 0) radius 115
  line L0 (0, 0) -> (10.0229, 114.5624)
  line L1 (0, 0) -> (73.9206, 88.0951)
  line L2 (0, 168) -> (0, -168) projected
  line L3 (0, 0) -> (76.014, 76.014)
  dimension "d92" = 215
  dimension "d93" = 4.3
  dimension "d96" = 360
  dimension "d98" = 200
  dimension "d99" = 230
  dimension "d101" = 5
  dimension "d102" = 5
  constraints: 10 centre point, 6 end point, 3 coincident, 2 point on circle, 1 vertical alignment, 19 other
  measures "d93" diameter of A1
  measures "d98" diameter of A9
  measures "d99" diameter of A10
  measures "d101" angle of L2 L0
  measures "d102" angle of L1 L3
sketch "Sketch5" plane through (0, 0, 14) normal (0, 0, 1) x (1, 0, 0)
  circle A0 centre (0, 0) radius 91
  circle A1 centre (0, 0) radius 65
  line L0 (0, 0) -> (6.3478, 90.7783)
  line L1 (0, 0) -> (32.2189, 56.453)
  line L2 (0, 168) -> (0, -168) projected
  circle A2 centre (6.3478, 90.7783) radius 2.1
  circle A3 centre (32.2189, 56.453) radius 2.1
  circle A4 centre (-67.0155, 61.5623) radius 2.1
  circle A5 centre (-89.9149, -14.0114) radius 2.1
  circle A6 centre (-45.1064, -79.0342) radius 2.1
  circle A7 centre (33.668, -84.5427) radius 2.1
  circle A8 centre (87.0898, -26.3888) radius 2.1
  circle A9 centre (74.9312, 51.6364) radius 2.1
  circle A10 centre (-24.0486, 60.3876) radius 2.1
  circle A11 centre (-62.207, 18.8491) radius 2.1
  circle A12 centre (-53.5223, -36.8832) radius 2.1
  circle A13 centre (-4.5342, -64.8417) radius 2.1
  circle A14 centre (47.8682, -43.9731) radius 2.1
  circle A15 centre (64.2249, 10.0081) radius 2.1
  dimension "d103" = 182
  dimension "d104" = 130
  dimension "d106" = 4
  dimension "d107" = 4.2
  dimension "d108" = 4.2
  dimension "d109" = 29.714
  dimension "d112" = 360
  dimension "d116" = 360
  constraints: 14 centre point, 4 coincident, 4 end point, 36 other
  measures "d106" angle of L2 L0
  measures "d107" diameter of A2
  measures "d108" diameter of A3
  measures "d109" angle of L2 L1
extrude "Extrusion6" cut sketch "Sketch5" against normal blind 8 contours A9 A0 | A0 A9 | A8 A0 | A0 A8 | A2 L0 A0 | A0 A2 | A7 A0 | A0 A7 | L0 A2 A0 | A3 A1 | A1 L1 A3 | A6 A0 | A0 A6 | A4 A0 | A0 A4 | A1 A3 L1 | A10 A1 | A1 A10 | A13 A1 | A1 A13 | A14 A1 | A1 A14 | A5 A0 | A0 A5 | A15 A1 | A1 A15 | A11 A1 | A1 A11 | A12 A1 | A1 A12
extrude "Extrusion7" cut sketch "Sketch4" against normal through all contours A0 A7 | A0 A7 | A8 L3 A0 | A0 A8 | A6 A0 | A0 A6 | L3 A8 A0 | A5 L2 A0 | A0 L2 A5 | L2 A5 A0 | A0 A5 L2 | A1 L2 A0 | A0 L2 A1 | A1 A0 L2 | A4 A0 | A0 A4 | A0 A1 L2 | A2 A0 | A0 A2 | A3 A0 | A0 A3
sketch "Sketch6" plane through (0, 0, 12) normal (0, 0, 1) x (1, 0, 0)
  circle A0 centre (0, 0) radius 120 projected
  line L0 (-120, 0) -> (-120, -120)
  line L1 (-120, -120) -> (120, -120)
  line L2 (120, -120) -> (120, 0)
  line L3 (-35, -114) -> (-85, -114)
  line L4 (-85, -114) -> (-85, -126)
  line L5 (-85, -126) -> (-35, -126)
  line L6 (-35, -126) -> (-35, -114)
  line L7 (-35, -114) -> (-85, -126) construction
  line L8 (-85, -114) -> (-35, -126) construction
  line L9 (35, -114) -> (85, -114)
  line L10 (85, -114) -> (85, -126)
  line L11 (85, -126) -> (35, -126)
  line L12 (35, -126) -> (35, -114)
  line L13 (35, -114) -> (85, -126) construction
  line L14 (85, -114) -> (35, -126) construction
  point P0 (-60, -120)
  point P1 (60, -120)
  point P2 (37.47, -114)
  point P3 (85, -120)
  point P4 (35, -120)
  point P5 (35, -114.7824)
  point P6 (0, -120)
  point P7 (-35, -114.7824)
  point P8 (-35, -120)
  point P9 (-85, -120)
  point P10 (-37.47, -114)
  dimension "d122" = 120
  dimension "d123" = 240
  dimension "d124" = 60
  dimension "d125" = 60
  dimension "d126" = 50
  dimension "d127" = 50
  dimension "d128" = 12
  dimension "d129" = 12
  constraints: 30 end point, 4 midpoint, 4 parallel, 3 perpendicular, 2 horizontal, 2 point on circle, 2 point on line, 2 tangent, 1 vertical
  measures "d122" distance of L0.start L0.end
  measures "d123" distance of L0.end L1.end
  measures "d124" distance from line of L2 point (60, -120)
  measures "d125" distance from line of L0 point (-60, -120)
  measures "d126" distance of L5.end L4.end
  measures "d127" distance of L10.end L11.end
  measures "d128" distance between parallel lines of L3 L5
  measures "d129" distance between parallel lines of L11 L9
extrude "Extrusion8" add sketch "Sketch6" against normal blind 12 contours L2 L1 L10 L9 A0 | A0 L3 L4 L1 L0 | L12 L1 A0 | A0 L1 L6
extrude "Extrusion9" cut sketch "Sketch6" against normal through all contours A0 L12 L9 | L3 L6 A0
fillet "Fillet1" radius 2 10 edges at (-120, -120, 6) (-85, -120, 6) (-85, -114, 6) (-35, -114, 6) (-35, -120, 6) (35, -120, 6) (35, -114, 6) (85, -114, 6) (85, -120, 6) (120, -120, 6)
sketch "Block2" plane through (0, 0, 0) normal (0, 0, 1) x (1, 0, 0)
  line L0 (83.1381, 5.88) -> (71.258, 5.88)
  line L1 (71.258, 5.88) -> (71.258, -6)
  line L2 (71.258, -6) -> (83.1381, -6)
  line L3 (83.1381, -6) -> (83.1381, 5.88)
  line L4 (83.1381, 5.88) -> (71.258, -6) construction
  line L5 (71.258, 5.88) -> (83.1381, -6) construction
  circle A0 centre (77.198, -0.06) radius 2
  circle A1 centre (72.671, -4.587) radius 2.1
  circle A2 centre (81.725, -4.587) radius 2.1
  circle A3 centre (81.725, 4.467) radius 2.1
  circle A4 centre (72.671, 4.467) radius 2.1
  circle A5 centre (70.898, -0.06) radius 0.75
  line L6 (70.898, -0.06) -> (77.198, -0.06)
  dimension "d9" = 11.88
  dimension "d11" = 4.2
  dimension "d17" = 360
  dimension "d18" = 142.521
  dimension "d19" = 0
  dimension "d20" = 45
  dimension "d21" = 90
  dimension "d22" = 135
  dimension "d23" = 180
  dimension "d24" = -45
  dimension "d25" = 90
  dimension "d26" = 135
  dimension "d27" = 180
  dimension "d28" = -45
  dimension "d29" = 90
  dimension "d30" = 135
  dimension "d31" = 0
  dimension "d32" = -45
  dimension "d33" = 90
  dimension "d34" = 45
  dimension "d35" = 140.97
  dimension "d36" = 360
  dimension "d37" = 0
  dimension "d38" = -32.727
  dimension "d8" = 11.88
  dimension "d10" = 4
  dimension "d12" = 1.413
  dimension "d13" = 360
  dimension "d14" = 1.5
  dimension "d15" = 6.3
  constraints: 6 end point, 2 centre point, 2 coincident, 2 midpoint, 1 horizontal, 1 point on line, 21 other
  measures "d8" distance of L5.end L4.end
  measures "d10" diameter of A0
  measures "d14" diameter of A5
  measures "d15" distance of L6.end L6.start
body "Solid1" dims "d61" = 157.40478, "d64" = 360 deg (derived), "d66" = 0, "d67" = -36 deg, "d68" = -72 deg, "d69" = -108 deg, "d70" = -144 deg, "d71" = -180 deg, "d72" = -216 deg, "d73" = -252 deg, "d74" = -288 deg, "d75" = -324 deg, "d76" = 0, "d77" = -36 deg, "d78" = -72 deg, "d79" = -108 deg, "d80" = -144 deg, "d81" = -180 deg, "d82" = -216 deg, "d83" = -252 deg, "d84" = -288 deg, "d85" = -324 deg
